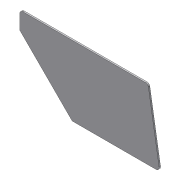
# Autodesk Inventor part: FE-00004-09
Saved by Autodesk Inventor 2012 (Build 160160000, 160)
## iProperties
Created: 2008-05-29
Part Number: FE-00004-09
Document SubType Name: Modeling
Designer: narosenberg
Density: 1 g/cm^3
Description: Plate, Shelf Support
Mass: 120.513 g
Surface Area: 785.03 cm^2
Volume: 120.513 cm^3
Material: Default
Author: narosenberg
Autodesk Inventor part; units mm, degrees
ref_plane "YZ Plane" through (0, 0, 0) normal (1, 0, 0) x (0, 1, 0)
ref_plane "XZ Plane" through (0, 0, 0) normal (0, 1, 0) x (-1, 0, 0)
ref_plane "XY Plane" through (0, 0, 0) normal (0, 0, 1) x (1, 0, 0)
sketch "Sketch1" plane through (0, 0, 0) normal (0, 0, 1) x (1, 0, 0)
  line L0 (-23.5242, 24.8428) -> (244.1465, 24.8428)
  line L1 (274.9258, 24.8428) -> (274.9258, -127.5572)
  line L2 (267.4299, -127.5572) -> (-29.8742, -127.5572)
  line L3 (-29.8742, -127.5572) -> (-29.8742, 18.4928)
  line L4 (250.4101, 19.5367) -> (273.6935, -120.1633)
  line L5 (-29.8742, -13.2572) -> (84.4258, -127.5572)
  arc A0 (-23.5242, 24.8428) -> (-29.8742, 18.4928) centre (-23.5242, 18.4928) ccw
  arc A1 (267.4299, -127.5572) -> (273.6935, -120.1633) centre (267.4299, -121.2072) ccw
  arc A2 (250.4101, 19.5367) -> (244.1465, 24.8428) centre (244.1465, 18.4928) ccw
  point P0 (-29.8742, 24.8428)
  point P1 (249.5258, 24.8428)
  dimension "d0" = 304.8
  dimension "d1" = 152.4
  dimension "d2" = 25.4
  dimension "d3" = 38.1
  dimension "d4" = 190.5
  dimension "d5" = 6.35
  dimension "d6" = 6.35
  constraints: 12 end point, 9 point on line, 6 point on circle, 6 tangent, 3 centre point, 2 parallel, 1 equal radius, 1 horizontal, 1 perpendicular
  measures "d0" distance of point (-29.874, 24.843) L1.start
  measures "d1" distance of L1.start L1.end
  measures "d2" distance of L1.start point (249.526, 24.843)
  measures "d3" distance of L5.start point (-29.874, 24.843)
  measures "d4" distance of L1.end L5.end
  measures "d5" radius of A0
  measures "d6" radius of A1
extrude "Extrusion1" add sketch "Sketch1" along normal blind 3.175 contours L0 A2 L4 A1 L2 L5 L3 A0
body "Solid1"
